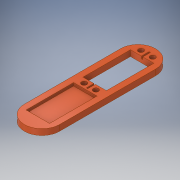
# Autodesk Inventor part: Femur_a
Saved by Autodesk Inventor 2017 (Build 210142000, 142)
## iProperties
Created: 2017-01-25
Part Number: Femur_a
Material: PET Plastic
Document SubType Name: Modeling
Designer: Alexander Miller
Density: 1.541 g/cm^3
Appearance: Smooth - Light Orange
Author: Alexander Miller
Autodesk Inventor part; units mm, degrees
ref_plane "YZ Plane" through (0, 0, 0) normal (1, 0, 0) x (0, 1, 0)
ref_plane "XZ Plane" through (0, 0, 0) normal (0, 1, 0) x (-1, 0, 0)
ref_plane "XY Plane" through (0, 0, 0) normal (0, 0, 1) x (1, 0, 0)
sketch "Sketch1" plane through (0, 0, 0) normal (0, 1, 0) x (-1, 0, 0)
  line L0 (-15, 56) -> (15, 56)
  line L1 (15, 56) -> (15, -56)
  line L2 (15, -56) -> (-15, -56)
  line L3 (-15, -56) -> (-15, 56)
  point P0 (0, 0)
  point P1 (15, 0)
  point P2 (0, 56)
  dimension "d0" = 30
  dimension "d1" = 112
  constraints: 8 end point, 2 midpoint, 2 parallel, 1 horizontal, 1 horizontal alignment, 1 perpendicular, 1 vertical alignment
  measures "d0" distance of L1.end L2.end
  measures "d1" distance of L0.end L1.end
extrude "Extrusion1" add sketch "Sketch1" along normal blind 5
sketch "Sketch2" plane through (0, 5, 0) normal (0, 1, 0) x (1, 0, 0)
  line L0 (10, 4) -> (-10, 4)
  line L1 (-10, 4) -> (-10, 44.5)
  line L2 (-10, 44.5) -> (10, 44.5)
  line L3 (10, 44.5) -> (10, 4)
  line L4 (-15, 56) -> (-15, -56) projected
  line L5 (15, 56) -> (-15, 56) projected
  line L6 (-21, 0) -> (21, 0) projected
  line L7 (10, -4) -> (-10, -4)
  line L8 (-10, -4) -> (-10, -44.5)
  line L9 (-10, -44.5) -> (10, -44.5)
  line L10 (10, -44.5) -> (10, -4)
  point P0 (0, 0)
  dimension "d4" = 5
  dimension "d5" = 20
  dimension "d6" = 40.5
  dimension "d7" = 11.5
  constraints: 16 end point, 4 symmetric about line, 2 parallel, 1 horizontal, 1 perpendicular
  measures "d4" distance between parallel lines of L1 L4
  measures "d5" distance of L1.end L2.end
  measures "d6" distance of L0.end L1.end
  measures "d7" distance between parallel lines of L5 L2
extrude "Extrusion2" cut sketch "Sketch2" against normal through all contours L0 L1 L2 L3
extrude "Extrusion3" cut sketch "Sketch2" against normal blind 2.5 contours L10 L9 L8 L7
sketch "Sketch3" plane through (0, 5, 0) normal (0, 1, 0) x (1, 0, 0)
  circle A0 centre (-5, 0) radius 2.25
  circle A1 centre (5, 0) radius 2.25
  circle A2 centre (-5, 48.5) radius 2.25
  circle A3 centre (5, 48.5) radius 2.25
  line L0 (15, 56) -> (-15, 56) projected
  line L1 (-10, 44.5) -> (10, 44.5) projected
  line L2 (10, 4) -> (-10, 4) projected
  line L3 (-10, 4) -> (-10, 44.5) projected
  line L4 (10, 44.5) -> (10, 4) projected
  point P0 (0, 0)
  dimension "d13" = 4
  dimension "d14" = 4
  dimension "d15" = 2.75
  dimension "d16" = 2.75
  dimension "d17" = 4.5
  constraints: 4 centre point, 3 equal radius, 2 horizontal alignment, 2 vertical alignment
  measures "d13" distance from line of L1 A2.centre
  measures "d14" distance from line of A0.centre L2
  measures "d15" distance edge to line of A2 L3
  measures "d16" distance edge to line of A3 L4
  measures "d17" diameter of A2
extrude "Extrusion4" cut sketch "Sketch3" against normal through all contours A0 | A1 | A2 | A3
sketch "Sketch4" plane through (0, 5, 0) normal (0, 1, 0) x (1, 0, 0)
  line L0 (-0.6, 4) -> (0.6, 4)
  line L1 (0.6, 4) -> (0.6, -2.5)
  line L2 (0.6, -2.5) -> (-0.6, -2.5)
  line L3 (-0.6, -2.5) -> (-0.6, 4)
  line L4 (-0.6, 44.5) -> (0.6, 44.5)
  line L5 (0.6, 44.5) -> (0.6, 51)
  line L6 (0.6, 51) -> (-0.6, 51)
  line L7 (-0.6, 51) -> (-0.6, 44.5)
  line L8 (10, 4) -> (-10, 4) projected
  line L9 (-10, 44.5) -> (10, 44.5) projected
  point P0 (0, 0)
  point P1 (0, 4)
  point P2 (0, 44.5)
  dimension "d20" = 6.5
  dimension "d21" = 1.2
  constraints: 16 end point, 4 parallel, 3 collinear, 2 horizontal, 2 midpoint, 2 perpendicular, 2 point on line, 2 vertical alignment
  measures "d20" distance of L6.end L4.start
  measures "d21" distance of L5.end L6.end
extrude "Extrusion5" cut sketch "Sketch4" against normal blind 2
full round fillet "Fillet1" first side at (15, 1.6667, -18.6667) centre faces at (-5, 1.6667, -56) second side at (-15, 1.6667, 18.6667)
full round fillet "Fillet2" first side at (-15, 1.6667, 23.6666) centre faces at (5, 1.6667, 56) second side at (15, 1.6667, -8.6667)
equation "\"d0\" = servo_depth + 2 * material_thickness"
equation "\"d1\" = -2 * servo_mount_hole_front_distance + 2 * servo_width + 4 * servo_mount_length + 2 * material_thickness"
equation "\"d2\" = material_thickness"
equation "\"d4\" = material_thickness"
equation "\"d5\" = servo_depth"
equation "\"d6\" = servo_width"
equation "\"d7\" = servo_mount_length + material_thickness"
equation "\"d8\" = material_thickness"
equation "\"d10\" = 0.5 * material_thickness"
equation "\"d13\" = servo_mount_length - servo_mount_hole_front_distance"
equation "\"d14\" = d13"
equation "\"d15\" = servo_mount_hole_side_distance"
equation "\"d16\" = d15"
equation "\"d17\" = servo_mount_hole_diameter"
equation "\"d18\" = 0.5 * material_thickness"
equation "\"d20\" = servo_mount_length"
equation "\"d21\" = servo_mount_pin_thickness"
equation "\"d22\" = servo_mount_pin_height"
equation "\"servo_depth\" = 20"
equation "\"material_thickness\" = 5"
equation "\"servo_mount_hole_front_distance\" = 2.5"
equation "\"servo_width\" = 40.5"
equation "\"servo_mount_length\" = 6.5"
equation "\"servo_mount_hole_side_distance\" = 2.75"
equation "\"servo_mount_hole_diameter\" = 4.5"
equation "\"servo_mount_pin_thickness\" = 1.2"
equation "\"servo_mount_pin_height\" = 2"
body "Solid1"
